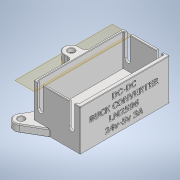
# Autodesk Inventor part: FAN PS CASE
Saved by Autodesk Inventor 2020 (Build 240168000, 168)
## iProperties
Created: 2019-12-23
Part Number: FAN PS CASE
Material: Generic
Document SubType Name: Modeling
Designer: pepd9
Density: 1 g/cm^3
Appearance: Default
Author: pepd9
Autodesk Inventor part; units mm, degrees
(part 1 of 2)
ref_plane "YZ Plane" through (0, 0, 0) normal (1, 0, 0) x (0, 1, 0)
ref_plane "XZ Plane" through (0, 0, 0) normal (0, 1, 0) x (-1, 0, 0)
ref_plane "XY Plane" through (0, 0, 0) normal (0, 0, 1) x (1, 0, 0)
sketch "Sketch1" plane through (0, 0, 0) normal (0, 1, 0) x (-1, 0, 0)
  line L0 (12.5, -25) -> (-12.5, -25)
  line L1 (-12.5, -25) -> (-12.5, 25)
  line L2 (-12.5, 25) -> (12.5, 25)
  line L3 (12.5, 25) -> (12.5, -25)
  line L4 (12.5, -25) -> (-12.5, 25) construction
  line L5 (-12.5, -25) -> (12.5, 25) construction
  line L6 (-12.5, -25) -> (-13.5, -25)
  line L7 (-13.5, -25) -> (-13.5, 25)
  line L8 (-13.5, 25) -> (-12.5, 25)
  line L9 (-12.5, 25) -> (-12.5, -25)
  point P0 (0, 0)
  point P1 (-13, 25)
  dimension "d6" = 25
  dimension "d7" = 50
  dimension "d98" = 1
  constraints: 20 end point, 4 parallel, 3 midpoint, 2 horizontal, 2 perpendicular, 1 horizontal alignment
  measures "d6" distance of L0.start L0.end
  measures "d7" distance of L0.end L1.end
  measures "d98" distance of L7.end L8.end
extrude "Extrusion1" add sketch "Sketch1" along normal blind 5
sketch "Sketch2" plane through (0, 5, 0) normal (0, 1, 0) x (1, 0, 0)
  point P0 (0, 0)
  point P1 (8, 15)
  point P2 (-8, -15)
  dimension "d2" = 30
  dimension "d3" = 16
  dimension "d4" = 8
  dimension "d5" = 15
  measures "d2" vertical distance of point (-8, -15) point (8, 15)
  measures "d3" horizontal distance of point (8, 15) point (-8, -15)
  measures "d4" horizontal distance of point (8, 15) point (0, 0)
  measures "d5" vertical distance of point (0, 0) point (8, 15)
hole "Hole1" at (8, 5, -15) at (-8, 5, 15) direction (0, -1, 0) diameter 3.4 end through all clearance for "Socket Head Cap Screw" size "M3" standard "Ansi Metric M Profile"
sketch "Sketch3" plane through (0, 0, 0) normal (0, -1, 0) x (1, 0, 0)
  circle A0 centre (-8, 15) radius 1.7 projected
  circle A1 centre (8, -15) radius 1.7 projected
  line L0 (-5.25, 13.4123) -> (-8, 11.8246)
  line L1 (-8, 11.8246) -> (-10.75, 13.4123)
  line L2 (-10.75, 13.4123) -> (-10.75, 16.5877)
  line L3 (-10.75, 16.5877) -> (-8, 18.1754)
  line L4 (-8, 18.1754) -> (-5.25, 16.5877)
  line L5 (-5.25, 16.5877) -> (-5.25, 13.4123)
  line L6 (10.75, -16.5877) -> (8, -18.1754)
  line L7 (8, -18.1754) -> (5.25, -16.5877)
  line L8 (5.25, -16.5877) -> (5.25, -13.4123)
  line L9 (5.25, -13.4123) -> (8, -11.8246)
  line L10 (8, -11.8246) -> (10.75, -13.4123)
  line L11 (10.75, -13.4123) -> (10.75, -16.5877)
  point P0 (0, 0)
  dimension "d15" = 5.5
  dimension "d16" = 5.5
  constraints: 24 end point, 2 coincident, 2 vertical, 26 other
  measures "d15" distance between parallel lines of L8 L11
  measures "d16" distance between parallel lines of L2 L5
extrude "Extrusion2" cut sketch "Sketch3" against normal blind 3
sketch "Sketch4" plane through (0, 5, 0) normal (0, 1, 0) x (1, 0, 0)
  circle A0 centre (8, 15) radius 1.7 projected
  circle A1 centre (-8, -15) radius 1.7 projected
  line L0 (-12.5, 25) -> (-12.5, -25) projected
  line L1 (-12.5, -25) -> (13.5, -25) projected
  circle A2 centre (8, 15) radius 1.7 projected
  circle A3 centre (8, 15) radius 3
  circle A4 centre (-8, -15) radius 3
  line L2 (13.5, 25) -> (-12.5, 25) projected
  line L3 (13.5, -25) -> (13.5, 25) projected
  point P0 (0, 0)
  dimension "d19" = 6
  dimension "d20" = 6
  constraints: 2 centre point, 2 coincident
  measures "d19" diameter of A3
  measures "d20" diameter of A4
extrude "Extrusion3" add sketch "Sketch4" along normal blind 4 contours A3 | A4
sketch "Sketch5" plane through (0, 3, 0) normal (0, -1, 0) x (1, 0, 0)
  line L0 (-5.25, 13.4123) -> (-8, 11.8246) projected
  line L1 (-5.25, 16.5877) -> (-5.25, 13.4123) projected
  line L2 (-8, 18.1754) -> (-5.25, 16.5877) projected
  line L3 (-10.75, 16.5877) -> (-8, 18.1754) projected
  line L4 (-10.75, 13.4123) -> (-10.75, 16.5877) projected
  line L5 (-8, 11.8246) -> (-10.75, 13.4123) projected
  circle A0 centre (-8, 15) radius 1.7 projected
  line L6 (10.75, -13.4123) -> (10.75, -16.5877) projected
  line L7 (8, -11.8246) -> (10.75, -13.4123) projected
  line L8 (5.25, -13.4123) -> (8, -11.8246) projected
  line L9 (5.25, -16.5877) -> (5.25, -13.4123) projected
  line L10 (8, -18.1754) -> (5.25, -16.5877) projected
  line L11 (10.75, -16.5877) -> (8, -18.1754) projected
  circle A1 centre (8, -15) radius 1.7 projected
  line L12 (-12.3859, 16.7) -> (-3.6141, 16.7)
  line L13 (-3.6141, 16.7) -> (-3.6141, 13.3)
  line L14 (-3.6141, 13.3) -> (-12.3859, 13.3)
  line L15 (-12.3859, 13.3) -> (-12.3859, 16.7)
  line L16 (-12.3859, 16.7) -> (-3.6141, 13.3) construction
  line L17 (-3.6141, 16.7) -> (-12.3859, 13.3) construction
  line L18 (4.5782, -13.3) -> (11.4218, -13.3)
  line L19 (11.4218, -13.3) -> (11.4218, -16.7)
  line L20 (11.4218, -16.7) -> (4.5782, -16.7)
  line L21 (4.5782, -16.7) -> (4.5782, -13.3)
  line L22 (4.5782, -13.3) -> (11.4218, -16.7) construction
  line L23 (11.4218, -13.3) -> (4.5782, -16.7) construction
  point P0 (0, 0)
  point P1 (5.4445, -16.7)
  point P2 (8, -16.7)
  point P3 (8, -13.3)
  point P4 (5.4445, -13.3)
  point P5 (10.5555, -13.3)
  point P6 (10.5555, -16.7)
  point P7 (-10.5555, 13.3)
  point P8 (-8, 13.3)
  point P9 (-8, 16.7)
  point P10 (-10.5555, 16.7)
  point P11 (-5.4445, 16.7)
  point P12 (-5.4445, 13.3)
  dimension "d23" = 3.4
  dimension "d24" = 3.4
  constraints: 24 end point, 4 midpoint, 4 parallel, 2 horizontal, 2 perpendicular
  measures "d23" distance of L12.end L13.end
  measures "d24" distance of L18.end L19.end
extrude "Extrusion4" cut sketch "Sketch5" against normal blind 0.5 contours L0 L14 A0 L12 L2 L1 | L14 L5 L4 L3 L12 A0 | L6 L11 L20 A1 L18 L7 | A1 L20 L10 L9 L8 L18
sketch "Sketch6" plane through (0, 3.5, 0) normal (0, -1, 0) x (1, 0, 0)
  line L0 (-5.25, 16.5877) -> (-5.25, 13.4123) projected
  line L1 (-5.4445, 16.7) -> (-5.25, 16.5877) projected
  line L2 (-8, 16.7) -> (-5.4445, 16.7) projected
  arc A0 (-8, 13.3) -> (-8, 16.7) centre (-8, 15) ccw projected
  line L3 (-5.4445, 13.3) -> (-8, 13.3) projected
  line L4 (-5.25, 13.4123) -> (-5.4445, 13.3) projected
  line L5 (-10.75, 16.5877) -> (-10.5555, 16.7) projected
  line L6 (-10.75, 13.4123) -> (-10.75, 16.5877) projected
  line L7 (-10.5555, 13.3) -> (-10.75, 13.4123) projected
  line L8 (-8, 13.3) -> (-10.5555, 13.3) projected
  arc A1 (-8, 16.7) -> (-8, 13.3) centre (-8, 15) ccw projected
  line L9 (-10.5555, 16.7) -> (-8, 16.7) projected
  line L10 (10.5555, -13.3) -> (10.75, -13.4123) projected
  line L11 (8, -13.3) -> (10.5555, -13.3) projected
  arc A2 (8, -16.7) -> (8, -13.3) centre (8, -15) ccw projected
  line L12 (10.5555, -16.7) -> (8, -16.7) projected
  line L13 (10.75, -16.5877) -> (10.5555, -16.7) projected
  line L14 (10.75, -13.4123) -> (10.75, -16.5877) projected
  line L15 (5.25, -13.4123) -> (5.4445, -13.3) projected
  line L16 (5.25, -16.5877) -> (5.25, -13.4123) projected
  line L17 (5.4445, -16.7) -> (5.25, -16.5877) projected
  line L18 (8, -16.7) -> (5.4445, -16.7) projected
  arc A3 (8, -13.3) -> (8, -16.7) centre (8, -15) ccw projected
  line L19 (5.4445, -13.3) -> (8, -13.3) projected
  line L20 (6.3, -12.0236) -> (9.7, -12.0236)
  line L21 (9.7, -12.0236) -> (9.7, -17.9764)
  line L22 (9.7, -17.9764) -> (6.3, -17.9764)
  line L23 (6.3, -17.9764) -> (6.3, -12.0236)
  line L24 (6.3, -12.0236) -> (9.7, -17.9764) construction
  line L25 (9.7, -12.0236) -> (6.3, -17.9764) construction
  line L26 (-9.7, 18.2149) -> (-6.3, 18.2149)
  line L27 (-6.3, 18.2149) -> (-6.3, 11.7851)
  line L28 (-6.3, 11.7851) -> (-9.7, 11.7851)
  line L29 (-9.7, 11.7851) -> (-9.7, 18.2149)
  line L30 (-9.7, 18.2149) -> (-6.3, 11.7851) construction
  line L31 (-6.3, 18.2149) -> (-9.7, 11.7851) construction
  point P0 (0, 0)
  point P1 (9.7, -16.7)
  point P2 (9.7, -15)
  point P3 (9.7, -13.3)
  point P4 (6.3, -13.3)
  point P5 (6.3, -15)
  point P6 (6.3, -16.7)
  point P7 (-9.7, 15)
  point P8 (-9.7, 13.3)
  point P9 (-9.7, 16.7)
  point P10 (-6.3, 15)
  point P11 (-6.3, 16.7)
  point P12 (-6.3, 13.3)
  dimension "d27" = 3.4
  dimension "d28" = 3.4
  constraints: 24 end point, 4 midpoint, 4 parallel, 2 horizontal, 2 perpendicular
  measures "d27" distance of L21.end L22.end
  measures "d28" distance of L27.end L28.end
extrude "Extrusion5" cut sketch "Sketch6" against normal blind 0.5 contours L27 A0 L2 | L3 A0 L27 | A1 L29 L9 | L8 L29 A1 | L21 A2 L11 | A3 L23 L19 | L21 L12 A2 | A3 L18 L23
sketch "Sketch7" plane through (0, 5, 0) normal (0, 1, 0) x (1, 0, 0)
  circle A0 centre (-8, -15) radius 3 projected
  circle A1 centre (8, 15) radius 3 projected
  line L0 (-12.5, 25) -> (-12.5, -25) projected
  line L1 (-12.5, -25) -> (13.5, -25) projected
  line L2 (11.3, 23.8) -> (11.3, -23.8)
  line L3 (11.3, -23.8) -> (-11.3, -23.8)
  line L4 (-11.3, -23.8) -> (-11.3, 23.8)
  line L5 (-11.3, 23.8) -> (11.3, 23.8)
  line L6 (13.5, 25) -> (-12.5, 25) projected
  line L7 (13.5, -25) -> (13.5, 25) projected
  point P0 (0, 0)
  constraints: 8 end point, 1 other
extrude "Extrusion6" add sketch "Sketch7" along normal blind 18 contours L6 L7 L1 L0
sketch "Sketch8" plane through (0, 0, 0) normal (0, -1, 0) x (1, 0, 0)
  circle A0 centre (-16.5, 28) radius 4
  circle A1 centre (-16.5, -12) radius 4
  line L0 (-12.5, -25) -> (-12.5, 25) projected
  line L1 (-12.5, 25) -> (13.5, 25) projected
  line L2 (-18.122, -15.6564) -> (-12.5, -18.9022)
  line L3 (-18.122, -8.3436) -> (-12.5, -5.0978)
  line L4 (-19.3561, 25.1995) -> (-12.5, 13.3244)
  line L5 (-14.0743, 31.1806) -> (-3.3692, 25)
  line L6 (-12.5, 25) -> (13.5, 25) projected
  point P0 (0, 0)
  point P1 (12.5, 25)
  point P2 (-12.5, -12)
  dimension "d34" = 8
  dimension "d35" = 8
  dimension "d36" = 4
  dimension "d37" = 40
  dimension "d38" = 3
  dimension "d39" = 60
  dimension "d40" = 60
  dimension "d41" = 30
  dimension "d42" = 30
  constraints: 8 end point, 4 point on circle, 4 point on line, 2 centre point, 1 vertical alignment
  measures "d34" diameter of A0
  measures "d35" diameter of A1
  measures "d36" distance from line of L0 A1.centre
  measures "d37" distance of A0.centre A1.centre
  measures "d38" distance from line of L1 A0.centre
  measures "d39" angle of L0 L2
  measures "d40" angle of L0 L3
  measures "d41" angle of L0 L4
  measures "d42" angle of L1 L5
extrude "Extrusion7" add sketch "Sketch8" against normal blind 4
sketch "Sketch9" plane through (0, 4, 0) normal (0, 1, 0) x (1, 0, 0)
  arc A0 (-18.122, 15.6564) -> (-18.122, 8.3436) centre (-16.5, 12) ccw projected
  arc A1 (-19.3561, -25.1995) -> (-14.0743, -31.1806) centre (-16.5, -28) ccw projected
  point P0 (0, 0)
hole "Hole2" at (-16.5, 4, -12) at (-16.5, 4, 28) direction (0, -1, 0) diameter 3.4 end through all clearance for "Socket Head Cap Screw" size "M3" standard "Ansi Metric M Profile"
sketch "Sketch10" plane through (12.5, 0, -25) normal (0, 0, -1) x (-1, 0, 0)
  line L0 (0, 0) -> (25, 0) projected
  line L1 (25, 0) -> (25, 23) projected
  line L2 (0, 23) -> (25, 23) projected
  line L3 (0, 0) -> (0, 23) projected
  circle A0 centre (3.75, 10.4995) radius 1.5
  circle A1 centre (21.25, 10.4995) radius 1.5
  line L4 (1.2, 23) -> (23.8, 23) projected
  line L5 (2.25, 10.4995) -> (5.25, 10.4995)
  line L6 (5.25, 10.4995) -> (5.25, 23)
  line L7 (5.25, 23) -> (2.25, 23)
  line L8 (2.25, 23) -> (2.25, 10.4995)
  line L9 (22.75, 10.4995) -> (19.75, 10.4995)
  line L10 (19.75, 10.4995) -> (19.75, 23)
  line L11 (19.75, 23) -> (22.75, 23)
  line L12 (22.75, 23) -> (22.75, 10.4995)
  point P0 (12.5, 0)
  point P1 (5.25, 10.4995)
  dimension "d52" = 3
  dimension "d53" = 3
  dimension "d54" = 3
  dimension "d72" = 3.75
  dimension "d73" = 3.75
  constraints: 16 end point, 4 parallel, 2 horizontal, 2 perpendicular, 2 point on line, 6 other
  measures "d54" distance of L10.end L11.end
  measures "d72" distance from line of L3 point (3.75, 10.499)
  measures "d73" distance from line of L1 point (21.25, 10.499)
extrude "Extrusion8" cut sketch "Sketch10" against normal through all contours L2 L6 A0 L8 | L12 A1 L10 L2 | L5 A0 | A0 L5 | L9 A1 | A1 L9
sketch "Sketch11" plane through (0, 0, 0) normal (0, -1, 0) x (1, 0, 0)
  circle A0 centre (-16.5, 0) radius 4
  line L0 (-12.5, -25) -> (-12.5, 25) projected
  line L1 (-12.5, 25) -> (13.5, 25) projected
  line L2 (-16.5, -4) -> (-12.5, -4)
  line L3 (-16.5, 4) -> (-12.5, 4)
  point P0 (0, 0)
  point P1 (-10.25, 25)
  dimension "d57" = 8
  dimension "d58" = 4
  dimension "d59" = 25
  constraints: 4 end point, 2 point on circle, 2 point on line, 2 tangent, 1 centre point, 1 horizontal, 1 perpendicular
  measures "d57" diameter of A0
  measures "d58" distance from line of A0.centre L0
  measures "d59" distance from line of L1 A0.centre
extrude "Extrusion9" add sketch "Sketch11" against normal up to surface (23 mm away)
sketch "Sketch12" plane through (0, 23, 0) normal (0, 1, 0) x (1, 0, 0)
  arc A0 (-16.5, 4) -> (-16.5, -4) centre (-16.5, 0) ccw projected
  point P0 (0, 0)
hole "Hole3" at (-16.5, 23, 0) direction (0, -1, 0) diameter 3.4 end through all clearance for "Socket Head Cap Screw" size "M3" standard "Ansi Metric M Profile"
sketch "Sketch13" plane through (0, 4, 0) normal (0, 1, 0) x (1, 0, 0)
  circle A0 centre (-16.5, 12) radius 1.7 projected
  line L0 (-18.122, 8.3436) -> (-12.5, 5.0978) projected
  line L1 (-12.5, 18.9022) -> (-12.5, 5.0978) projected
  line L2 (-12.5, 18.9022) -> (-18.122, 15.6564) projected
  arc A1 (-18.122, 15.6564) -> (-18.122, 8.3436) centre (-16.5, 12) ccw projected
  circle A2 centre (-16.5, 0) radius 1.7 projected
  line L3 (-12.5, 25) -> (-12.5, 4) projected
  line L4 (-16.5, 4) -> (-12.5, 4) projected
  arc A3 (-16.5, 4) -> (-16.5, -4) centre (-16.5, 0) ccw projected
  line L5 (-12.5, -4) -> (-16.5, -4) projected
  line L6 (-12.5, -4) -> (-12.5, -25) projected
  line L7 (-12.5, -25) -> (-10.25, -25) projected
  line L8 (-10.25, -23.8) -> (-11.3, -23.8) projected
  line L9 (-11.3, -23.8) -> (-11.3, 23.8) projected
  line L10 (-11.3, 23.8) -> (-10.25, 23.8) projected
  arc A4 (-18.122, 15.6564) -> (-18.122, 8.3436) centre (-16.5, 12) ccw projected
  line L11 (-20.5, 12) -> (-20.5, 0)
  line L12 (13.5, -25) -> (13.5, 25) projected
  line L13 (7.25, 25) -> (-7.25, 25) projected
  line L14 (11.3, 23.8) -> (11.3, -23.8) projected
  line L15 (-10.25, 23.8) -> (-10.25, 25) projected
  line L16 (-10.25, 25) -> (-12.5, 25) projected
  line L17 (-10.25, -25) -> (-10.25, -23.8) projected
  line L18 (-7.25, 25) -> (-7.25, 23.8) projected
  line L19 (-7.25, 23.8) -> (7.25, 23.8) projected
  line L20 (7.25, 23.8) -> (7.25, 25) projected
  line L21 (10.25, 25) -> (10.25, 23.8) projected
  line L22 (10.25, 23.8) -> (11.3, 23.8) projected
  line L23 (11.3, -23.8) -> (10.25, -23.8) projected
  line L24 (10.25, -23.8) -> (10.25, -25) projected
  line L25 (10.25, -25) -> (13.5, -25) projected
  line L26 (13.5, 25) -> (10.25, 25) projected
  point P0 (0, 0)
  constraints: 3 point on circle, 2 end point
extrude "Extrusion10" add sketch "Sketch13" against normal up to surface (4 mm away) contours L0 L3 L4 A3 L11 A1
fillet "Fillet1" radius 2 2 edges at (-12.5, 11.5, 4) (-12.5, 13.5, -4)
fillet "Fillet2" radius 0.4 12 edges at (11.3, 14, -23.8) (-11.3, 14, -23.8) (11.3, 14, 23.8) (-11.3, 14, 23.8) (-12.5, 13.5, 25) (-3.3692, 2, 25) (-12.5, 2, 13.3244) (-12.5, 2, -18.9022) (-19.3561, 2, 25.1995) (13.5, 11.5, -25) (-12.5, 11.5, -25) (13.5, 11.5, 25)
chamfer "Chamfer1" distance 0.6 angle 45 12 edges at (5.25, 0, -15) (6.625, 0, -17.3816) (9.375, 0, -17.3816) (10.75, 0, -15) (9.375, 0, -12.6184) (6.625, 0, -12.6184) (-10.75, 0, 15) (-9.375, 0, 12.6184) (-6.625, 0, 12.6184) (-5.25, 0, 15) (-6.625, 0, 17.3816) (-9.375, 0, 17.3816)
chamfer "Chamfer2" distance 0.5 angle 45 10 edges at (-19.4826, 4, 30.6653) (-19.3578, 4, 25.1967) (-15.9425, 4, 19.287) (-12.5136, 4, 13.3208) (-8.7682, 4, 28.1171) (-3.3656, 4, 25.0136) (-20.5, 4, -6) (-19.8532, 4, -14.1808) (-15.411, 4, -17.2216) (-12.5536, 4, -18.9332)
chamfer "Chamfer3" distance 0.25 angle 45 26 edges at (-16.5, 4, -13.7) (-16.5, 4, 26.3) (-20.5, 23, 0) (-15.5, 23, -4) (-13.0858, 23, -4.5858) (-12.5, 23, 15.3) (-12.5, 23, -15.3) (-15.5, 23, 4) (-13.0858, 23, 4.5858) (-12.3828, 23, 24.8828) (-11.175, 23, 25) (-16.5, 23, -1.7) (0, 23, 25) (11.675, 23, 25) (11.3, 23, 0) (11.1828, 23, 23.6828) (10.575, 23, 23.8) (11.1828, 23, -23.6828) (10.575, 23, -23.8) (0, 23, 23.8) (0, 23, -23.8) (-11.3, 23, 0) (-11.1828, 23, -23.6828) (-10.575, 23, -23.8) (-11.1828, 23, 23.6828) (-10.575, 23, 23.8)
ref_plane "Work Plane1" through (0, 20, 0) normal (0, 1, 0) x (1, 0, 0)
sketch "Sketch14" plane through (0, 20, 0) normal (0, 1, 0) x (1, 0, 0)
  circle A0 centre (-16.5, 0) radius 1.7 projected
  line L0 (-19.4, -2.85) -> (-13.6, -2.85)
  line L1 (-13.6, -2.85) -> (-13.6, 2.85)
  line L2 (-13.6, 2.85) -> (-19.4, 2.85)
  line L3 (-19.4, 2.85) -> (-19.4, -2.85)
  line L4 (-19.4, -2.85) -> (-13.6, 2.85) construction
  line L5 (-13.6, -2.85) -> (-19.4, 2.85) construction
  line L6 (-19.4, -2.85) -> (-24.9, -2.85)
  line L7 (-24.9, -2.85) -> (-24.9, 2.85)
  line L8 (-24.9, 2.85) -> (-19.4, 2.85)
  line L9 (-19.4, 2.85) -> (-19.4, -2.85)
  point P0 (0, 0)
  dimension "d85" = 5.8
  dimension "d86" = 5.7
  dimension "d87" = 5.5
  dimension "d88" = 5.7
  constraints: 20 end point, 4 parallel, 2 horizontal, 2 midpoint, 2 perpendicular
  measures "d85" distance of L2.end L1.end
  measures "d86" distance of L1.end L0.end
  measures "d87" distance of L7.end L8.end
  measures "d88" distance of L6.end L7.end
extrude "Extrusion11" cut sketch "Sketch14" against normal blind 1.7
sketch "Sketch15" plane through (0, 20, 0) normal (0, -1, 0) x (1, 0, 0)
  arc A0 (-19.3067, 2.85) -> (-19.3067, -2.85) centre (-16.5, 0) ccw projected
  line L0 (-13.6, -2.85) -> (-19.3067, -2.85) projected
  line L1 (-13.6, 2.85) -> (-13.6, -2.85) projected
  line L2 (-19.3067, 2.85) -> (-13.6, 2.85) projected
  circle A1 centre (-16.5, 0) radius 1.7 projected
  line L3 (-14.8283, -3.0472) -> (-18.2283, -3.0472)
  line L4 (-18.2283, -3.0472) -> (-18.2283, 3.0472)
  line L5 (-18.2283, 3.0472) -> (-14.8283, 3.0472)
  line L6 (-14.8283, 3.0472) -> (-14.8283, -3.0472)
  line L7 (-14.8283, -3.0472) -> (-18.2283, 3.0472) construction
  line L8 (-18.2283, -3.0472) -> (-14.8283, 3.0472) construction
  point P0 (0, 0)
  point P1 (-16.5283, 0)
  point P2 (-14.8283, -2.85)
  point P3 (-14.8283, -0.3088)
  point P4 (-14.8283, 0.3088)
  point P5 (-14.8283, 2.85)
  point P6 (-18.2283, 2.85)
  point P7 (-18.2283, -2.85)
  dimension "d91" = 3.4
  constraints: 12 end point, 2 midpoint, 2 parallel, 1 horizontal, 1 perpendicular
  measures "d91" distance of L4.end L5.end
extrude "Extrusion12" cut sketch "Sketch15" against normal blind 0.5 contours L2 L6 A1 L0 L4
sketch "Sketch16" plane through (0, 20.5, 0) normal (0, -1, 0) x (1, 0, 0)
  arc A0 (-14.8283, 0.3088) -> (-14.8283, -0.3088) centre (-16.5, 0) ccw projected
  line L0 (-14.8, -1.7) -> (-18.2, -1.7)
  line L1 (-18.2, -1.7) -> (-18.2, 1.7)
  line L2 (-18.2, 1.7) -> (-14.8, 1.7)
  line L3 (-14.8, 1.7) -> (-14.8, -1.7)
  line L4 (-14.8, -1.7) -> (-18.2, 1.7) construction
  line L5 (-18.2, -1.7) -> (-14.8, 1.7) construction
  circle A1 centre (-16.5, 0) radius 1.7 projected
  point P0 (0, 0)
  point P1 (-14.8, 0)
  point P2 (-16.5, 1.7)
  point P3 (-16.5, -1.7)
  point P4 (-18.2, 0)
  dimension "d94" = 3.4
  dimension "d95" = 3.4
  constraints: 12 end point, 2 midpoint, 2 parallel, 1 horizontal, 1 perpendicular
  measures "d94" distance of L1.end L2.end
  measures "d95" distance of L0.end L1.end
extrude "Extrusion13" cut sketch "Sketch16" against normal blind 0.5 contours A0 L2 L3 A1 | A0 L1 L2 | L3 L0 A0 A1 | A0 L0 L1
sketch "Sketch17" plane through (13.5, 0.25, 24.6) normal (1, 0, 0) x (0, 0, -1)
  line L0 (4.6127, 20.5668) -> (43.452, 20.5668) construction
  line L1 (43.452, 20.5668) -> (43.452, 2.328) construction
  line L2 (43.452, 2.328) -> (4.6127, 2.328) construction
  line L3 (4.6127, 2.328) -> (4.6127, 20.5668) construction
  spline S0 degree 2 poles (20.189, 18.98) (20.189, 18.5524) (19.8158, 17.8801) (19.5315, 17.6997) knots 0 0 0 1 2 2 2
  spline S1 degree 2 poles (19.5315, 17.6997) (19.2942, 17.5465) (18.7356, 17.4575) (18.4217, 17.4575) knots 0 0 0 1 2 2 2
  line L4 (18.4217, 17.4575) -> (17.4677, 17.4575)
  line L5 (17.4677, 17.4575) -> (17.4677, 20.5075)
  line L6 (17.4677, 20.5075) -> (18.4119, 20.5075)
  spline S2 degree 2 poles (18.4119, 20.5075) (18.7332, 20.5075) (19.2942, 20.4259) (19.5414, 20.2677) knots 0 0 0 1 2 2 2
  spline S3 degree 2 poles (19.5414, 20.2677) (19.8405, 20.0749) (20.189, 19.4224) (20.189, 18.98) knots 0 0 0 1 2 2 2
  spline S4 degree 2 poles (19.403, 18.985) (19.403, 19.2865) (19.1954, 19.7166) (18.9828, 19.8377) knots 0 0 0 1 2 2 2
  spline S5 degree 2 poles (18.9828, 19.8377) (18.8271, 19.9217) (18.486, 19.939) (18.2487, 19.939) knots 0 0 0 1 2 2 2
  line L7 (18.2487, 19.939) -> (18.2339, 19.939)
  line L8 (18.2339, 19.939) -> (18.2339, 18.0284)
  line L9 (18.2339, 18.0284) -> (18.2487, 18.0284)
  spline S6 degree 2 poles (18.2487, 18.0284) (18.5058, 18.0284) (18.8592, 18.0457) (19.0199, 18.1471) knots 0 0 0 1 2 2 2
  spline S7 degree 2 poles (19.0199, 18.1471) (19.2077, 18.2657) (19.403, 18.6834) (19.403, 18.985) knots 0 0 0 1 2 2 2
  spline S8 degree 2 poles (21.9587, 17.3982) (21.2715, 17.3982) (20.4658, 18.2286) (20.4658, 18.98) knots 0 0 0 1 2 2 2
  spline S9 degree 2 poles (20.4658, 18.98) (20.4658, 19.7042) (21.274, 20.5668) (21.9611, 20.5668) knots 0 0 0 1 2 2 2
  spline S10 degree 2 poles (21.9611, 20.5668) (22.1416, 20.5668) (22.4332, 20.5248) (22.5667, 20.4902) knots 0 0 0 1 2 2 2
  spline S11 degree 2 poles (22.5667, 20.4902) (22.6705, 20.4581) (22.9152, 20.3518) (22.9918, 20.3122) knots 0 0 0 1 2 2 2
  line L10 (22.9918, 20.3122) -> (22.9918, 19.5856)
  line L11 (22.9918, 19.5856) -> (22.9152, 19.5856)
  spline S12 degree 2 poles (22.9152, 19.5856) (22.8583, 19.635) (22.6903, 19.7734) (22.584, 19.8377) knots 0 0 0 1 2 2 2
  spline S13 degree 2 poles (22.584, 19.8377) (22.4777, 19.9044) (22.2231, 19.9959) (22.0822, 19.9959) knots 0 0 0 1 2 2 2
  spline S14 degree 2 poles (22.0822, 19.9959) (21.9166, 19.9959) (21.6423, 19.892) (21.5162, 19.761) knots 0 0 0 1 2 2 2
  spline S15 degree 2 poles (21.5162, 19.761) (21.4025, 19.6449) (21.2567, 19.2469) (21.2567, 18.9775) knots 0 0 0 1 2 2 2
  spline S16 degree 2 poles (21.2567, 18.9775) (21.2567, 18.6933) (21.4075, 18.3053) (21.5311, 18.1866) knots 0 0 0 1 2 2 2
  spline S17 degree 2 poles (21.5311, 18.1866) (21.6497, 18.0704) (21.9414, 17.9691) (22.0872, 17.9691) knots 0 0 0 1 2 2 2
  spline S18 degree 2 poles (22.0872, 17.9691) (22.238, 17.9691) (22.5123, 18.0704) (22.6062, 18.1322) knots 0 0 0 1 2 2 2
  spline S19 degree 2 poles (22.6062, 18.1322) (22.71, 18.194) (22.8658, 18.325) (22.9226, 18.3769) knots 0 0 0 1 2 2 2
  line L12 (22.9226, 18.3769) -> (22.9918, 18.3769)
  line L13 (22.9918, 18.3769) -> (22.9918, 17.6602)
  spline S20 degree 2 poles (22.9918, 17.6602) (22.9078, 17.6206) (22.6878, 17.5217) (22.5692, 17.4871) knots 0 0 0 1 2 2 2
  spline S21 degree 2 poles (22.5692, 17.4871) (22.4258, 17.4427) (22.1762, 17.3982) (21.9587, 17.3982) knots 0 0 0 1 2 2 2
  line L14 (24.7096, 18.5203) -> (23.3527, 18.5203)
  line L15 (23.3527, 18.5203) -> (23.3527, 19.0888)
  line L16 (23.3527, 19.0888) -> (24.7096, 19.0888)
  line L17 (24.7096, 19.0888) -> (24.7096, 18.5203)
  spline S22 degree 2 poles (27.9746, 18.98) (27.9746, 18.5524) (27.6014, 17.8801) (27.3172, 17.6997) knots 0 0 0 1 2 2 2
  spline S23 degree 2 poles (27.3172, 17.6997) (27.0799, 17.5465) (26.5213, 17.4575) (26.2074, 17.4575) knots 0 0 0 1 2 2 2
  line L18 (26.2074, 17.4575) -> (25.2534, 17.4575)
  line L19 (25.2534, 17.4575) -> (25.2534, 20.5075)
  line L20 (25.2534, 20.5075) -> (26.1975, 20.5075)
  spline S24 degree 2 poles (26.1975, 20.5075) (26.5188, 20.5075) (27.0799, 20.4259) (27.3271, 20.2677) knots 0 0 0 1 2 2 2
  spline S25 degree 2 poles (27.3271, 20.2677) (27.6261, 20.0749) (27.9746, 19.4224) (27.9746, 18.98) knots 0 0 0 1 2 2 2
  spline S26 degree 2 poles (27.1886, 18.985) (27.1886, 19.2865) (26.981, 19.7166) (26.7685, 19.8377) knots 0 0 0 1 2 2 2
  spline S27 degree 2 poles (26.7685, 19.8377) (26.6128, 19.9217) (26.2717, 19.939) (26.0344, 19.939) knots 0 0 0 1 2 2 2
  line L21 (26.0344, 19.939) -> (26.0196, 19.939)
  line L22 (26.0196, 19.939) -> (26.0196, 18.0284)
  line L23 (26.0196, 18.0284) -> (26.0344, 18.0284)
  spline S28 degree 2 poles (26.0344, 18.0284) (26.2914, 18.0284) (26.6449, 18.0457) (26.8055, 18.1471) knots 0 0 0 1 2 2 2
  spline S29 degree 2 poles (26.8055, 18.1471) (26.9934, 18.2657) (27.1886, 18.6834) (27.1886, 18.985) knots 0 0 0 1 2 2 2
  spline S30 degree 2 poles (29.7443, 17.3982) (29.0572, 17.3982) (28.2514, 18.2286) (28.2514, 18.98) knots 0 0 0 1 2 2 2
  spline S31 degree 2 poles (28.2514, 18.98) (28.2514, 19.7042) (29.0597, 20.5668) (29.7468, 20.5668) knots 0 0 0 1 2 2 2
  spline S32 degree 2 poles (29.7468, 20.5668) (29.9272, 20.5668) (30.2189, 20.5248) (30.3523, 20.4902) knots 0 0 0 1 2 2 2
  spline S33 degree 2 poles (30.3523, 20.4902) (30.4561, 20.4581) (30.7008, 20.3518) (30.7775, 20.3122) knots 0 0 0 1 2 2 2
  line L24 (30.7775, 20.3122) -> (30.7775, 19.5856)
  line L25 (30.7775, 19.5856) -> (30.7008, 19.5856)
  spline S34 degree 2 poles (30.7008, 19.5856) (30.644, 19.635) (30.4759, 19.7734) (30.3696, 19.8377) knots 0 0 0 1 2 2 2
  spline S35 degree 2 poles (30.3696, 19.8377) (30.2634, 19.9044) (30.0088, 19.9959) (29.8679, 19.9959) knots 0 0 0 1 2 2 2
  spline S36 degree 2 poles (29.8679, 19.9959) (29.7023, 19.9959) (29.4279, 19.892) (29.3019, 19.761) knots 0 0 0 1 2 2 2
  spline S37 degree 2 poles (29.3019, 19.761) (29.1882, 19.6449) (29.0424, 19.2469) (29.0424, 18.9775) knots 0 0 0 1 2 2 2
  spline S38 degree 2 poles (29.0424, 18.9775) (29.0424, 18.6933) (29.1931, 18.3053) (29.3167, 18.1866) knots 0 0 0 1 2 2 2
  spline S39 degree 2 poles (29.3167, 18.1866) (29.4354, 18.0704) (29.727, 17.9691) (29.8728, 17.9691) knots 0 0 0 1 2 2 2
  spline S40 degree 2 poles (29.8728, 17.9691) (30.0236, 17.9691) (30.298, 18.0704) (30.3919, 18.1322) knots 0 0 0 1 2 2 2
  spline S41 degree 2 poles (30.3919, 18.1322) (30.4957, 18.194) (30.6514, 18.325) (30.7083, 18.3769) knots 0 0 0 1 2 2 2
  line L26 (30.7083, 18.3769) -> (30.7775, 18.3769)
  line L27 (30.7775, 18.3769) -> (30.7775, 17.6602)
  spline S42 degree 2 poles (30.7775, 17.6602) (30.6934, 17.6206) (30.4735, 17.5217) (30.3548, 17.4871) knots 0 0 0 1 2 2 2
  spline S43 degree 2 poles (30.3548, 17.4871) (30.2115, 17.4427) (29.9618, 17.3982) (29.7443, 17.3982) knots 0 0 0 1 2 2 2
  spline S44 degree 2 poles (7.3661, 13.37) (7.3661, 13.1426) (7.1931, 12.7991) (7.0497, 12.6854) knots 0 0 0 1 2 2 2
  spline S45 degree 2 poles (7.0497, 12.6854) (6.8767, 12.5494) (6.4664, 12.4357) (6.1476, 12.4357) knots 0 0 0 1 2 2 2
  line L28 (6.1476, 12.4357) -> (4.9291, 12.4357)
  line L29 (4.9291, 12.4357) -> (4.9291, 15.4857)
  line L30 (4.9291, 15.4857) -> (6.0042, 15.4857)
  spline S46 degree 2 poles (6.0042, 15.4857) (6.3404, 15.4857) (6.6864, 15.4338) (6.8372, 15.3523) knots 0 0 0 1 2 2 2
  spline S47 degree 2 poles (6.8372, 15.3523) (7.0028, 15.2658) (7.1634, 14.9692) (7.1634, 14.7764) knots 0 0 0 1 2 2 2
  spline S48 degree 2 poles (7.1634, 14.7764) (7.1634, 14.5539) (6.941, 14.2054) (6.7433, 14.1239) knots 0 0 0 1 2 2 2
  line L31 (6.7433, 14.1239) -> (6.7433, 14.109)
  spline S49 degree 2 poles (6.7433, 14.109) (7.0275, 14.0497) (7.3661, 13.6814) (7.3661, 13.37) knots 0 0 0 1 2 2 2
  spline S50 degree 2 poles (6.5752, 13.3824) (6.5752, 13.5257) (6.4615, 13.6864) (6.3478, 13.7284) knots 0 0 0 1 2 2 2
  spline S51 degree 2 poles (6.3478, 13.7284) (6.2786, 13.7556) (6.0339, 13.7605) (5.8312, 13.7605) knots 0 0 0 1 2 2 2
  line L32 (5.8312, 13.7605) -> (5.6903, 13.7605)
  line L33 (5.6903, 13.7605) -> (5.6903, 12.9919)
  line L34 (5.6903, 12.9919) -> (5.7324, 12.9919)
  spline S52 degree 2 poles (5.7324, 12.9919) (6.029, 12.9919) (6.2564, 12.9993) (6.375, 13.0512) knots 0 0 0 1 2 2 2
  spline S53 degree 2 poles (6.375, 13.0512) (6.4788, 13.0981) (6.5752, 13.2712) (6.5752, 13.3824) knots 0 0 0 1 2 2 2
  spline S54 degree 2 poles (6.3849, 14.6256) (6.3849, 14.6998) (6.3083, 14.8555) (6.2292, 14.8901) knots 0 0 0 1 2 2 2
  spline S55 degree 2 poles (6.2292, 14.8901) (6.155, 14.9247) (5.9474, 14.9296) (5.7423, 14.9296) knots 0 0 0 1 2 2 2
  line L35 (5.7423, 14.9296) -> (5.6903, 14.9296)
  line L36 (5.6903, 14.9296) -> (5.6903, 14.2821)
  line L37 (5.6903, 14.2821) -> (5.7867, 14.2821)
  spline S56 degree 2 poles (5.7867, 14.2821) (5.982, 14.2821) (6.1402, 14.2895) (6.2242, 14.329) knots 0 0 0 1 2 2 2
  spline S57 degree 2 poles (6.2242, 14.329) (6.3157, 14.3735) (6.3849, 14.5243) (6.3849, 14.6256) knots 0 0 0 1 2 2 2
  spline S58 degree 2 poles (9.0394, 12.3715) (8.424, 12.3715) (7.7616, 12.9647) (7.7616, 13.5381) knots 0 0 0 1 2 2 2
  line L38 (7.7616, 13.5381) -> (7.7616, 15.4857)
  line L39 (7.7616, 15.4857) -> (8.5278, 15.4857)
  line L40 (8.5278, 15.4857) -> (8.5278, 13.5826)
  spline S59 degree 2 poles (8.5278, 13.5826) (8.5278, 13.2637) (8.7675, 12.9523) (9.0394, 12.9523) knots 0 0 0 1 2 2 2
  spline S60 degree 2 poles (9.0394, 12.9523) (9.3039, 12.9523) (9.551, 13.2514) (9.551, 13.5826) knots 0 0 0 1 2 2 2
  line L41 (9.551, 13.5826) -> (9.551, 15.4857)
  line L42 (9.551, 15.4857) -> (10.3173, 15.4857)
  line L43 (10.3173, 15.4857) -> (10.3173, 13.5406)
  spline S61 degree 2 poles (10.3173, 13.5406) (10.3173, 12.977) (9.6722, 12.3715) (9.0394, 12.3715) knots 0 0 0 1 2 2 2
  spline S62 degree 2 poles (12.2204, 12.3764) (11.5333, 12.3764) (10.7275, 13.2069) (10.7275, 13.9583) knots 0 0 0 1 2 2 2
  spline S63 degree 2 poles (10.7275, 13.9583) (10.7275, 14.6825) (11.5358, 15.5451) (12.2229, 15.5451) knots 0 0 0 1 2 2 2
  spline S64 degree 2 poles (12.2229, 15.5451) (12.4033, 15.5451) (12.695, 15.503) (12.8284, 15.4684) knots 0 0 0 1 2 2 2
  spline S65 degree 2 poles (12.8284, 15.4684) (12.9322, 15.4363) (13.1769, 15.33) (13.2536, 15.2905) knots 0 0 0 1 2 2 2
  line L44 (13.2536, 15.2905) -> (13.2536, 14.5638)
  line L45 (13.2536, 14.5638) -> (13.1769, 14.5638)
  spline S66 degree 2 poles (13.1769, 14.5638) (13.1201, 14.6133) (12.952, 14.7517) (12.8457, 14.8159) knots 0 0 0 1 2 2 2
  spline S67 degree 2 poles (12.8457, 14.8159) (12.7395, 14.8827) (12.4849, 14.9741) (12.344, 14.9741) knots 0 0 0 1 2 2 2
  spline S68 degree 2 poles (12.344, 14.9741) (12.1784, 14.9741) (11.904, 14.8703) (11.778, 14.7393) knots 0 0 0 1 2 2 2
  spline S69 degree 2 poles (11.778, 14.7393) (11.6643, 14.6231) (11.5185, 14.2252) (11.5185, 13.9558) knots 0 0 0 1 2 2 2
  spline S70 degree 2 poles (11.5185, 13.9558) (11.5185, 13.6716) (11.6692, 13.2835) (11.7928, 13.1649) knots 0 0 0 1 2 2 2
  spline S71 degree 2 poles (11.7928, 13.1649) (11.9115, 13.0487) (12.2031, 12.9474) (12.3489, 12.9474) knots 0 0 0 1 2 2 2
  spline S72 degree 2 poles (12.3489, 12.9474) (12.4997, 12.9474) (12.7741, 13.0487) (12.868, 13.1105) knots 0 0 0 1 2 2 2
  spline S73 degree 2 poles (12.868, 13.1105) (12.9718, 13.1723) (13.1275, 13.3033) (13.1843, 13.3552) knots 0 0 0 1 2 2 2
  line L46 (13.1843, 13.3552) -> (13.2536, 13.3552)
  line L47 (13.2536, 13.3552) -> (13.2536, 12.6384)
  spline S74 degree 2 poles (13.2536, 12.6384) (13.1695, 12.5989) (12.9495, 12.5) (12.8309, 12.4654) knots 0 0 0 1 2 2 2
  spline S75 degree 2 poles (12.8309, 12.4654) (12.6876, 12.4209) (12.4379, 12.3764) (12.2204, 12.3764) knots 0 0 0 1 2 2 2
  line L48 (16.3777, 12.4357) -> (15.4508, 12.4357)
  line L49 (15.4508, 12.4357) -> (14.6228, 13.674)
  line L50 (14.6228, 13.674) -> (14.4721, 13.4664)
  line L51 (14.4721, 13.4664) -> (14.4721, 12.4357)
  line L52 (14.4721, 12.4357) -> (13.7059, 12.4357)
  line L53 (13.7059, 12.4357) -> (13.7059, 15.4857)
  line L54 (13.7059, 15.4857) -> (14.4721, 15.4857)
  line L55 (14.4721, 15.4857) -> (14.4721, 14.1239)
  line L56 (14.4721, 14.1239) -> (15.4508, 15.4857)
  line L57 (15.4508, 15.4857) -> (16.3332, 15.4857)
  line L58 (16.3332, 15.4857) -> (15.2457, 14.0695)
  line L59 (15.2457, 14.0695) -> (16.3777, 12.4357)
  spline S76 degree 2 poles (19.1707, 12.3764) (18.4835, 12.3764) (17.6778, 13.2069) (17.6778, 13.9583) knots 0 0 0 1 2 2 2
  spline S77 degree 2 poles (17.6778, 13.9583) (17.6778, 14.6825) (18.486, 15.5451) (19.1731, 15.5451) knots 0 0 0 1 2 2 2
  spline S78 degree 2 poles (19.1731, 15.5451) (19.3536, 15.5451) (19.6452, 15.503) (19.7787, 15.4684) knots 0 0 0 1 2 2 2
  spline S79 degree 2 poles (19.7787, 15.4684) (19.8825, 15.4363) (20.1272, 15.33) (20.2038, 15.2905) knots 0 0 0 1 2 2 2
  line L60 (20.2038, 15.2905) -> (20.2038, 14.5638)
  line L61 (20.2038, 14.5638) -> (20.1272, 14.5638)
  spline S80 degree 2 poles (20.1272, 14.5638) (20.0703, 14.6133) (19.9023, 14.7517) (19.796, 14.8159) knots 0 0 0 1 2 2 2
  spline S81 degree 2 poles (19.796, 14.8159) (19.6897, 14.8827) (19.4351, 14.9741) (19.2942, 14.9741) knots 0 0 0 1 2 2 2
  spline S82 degree 2 poles (19.2942, 14.9741) (19.1286, 14.9741) (18.8543, 14.8703) (18.7282, 14.7393) knots 0 0 0 1 2 2 2
  spline S83 degree 2 poles (18.7282, 14.7393) (18.6145, 14.6231) (18.4687, 14.2252) (18.4687, 13.9558) knots 0 0 0 1 2 2 2
  spline S84 degree 2 poles (18.4687, 13.9558) (18.4687, 13.6716) (18.6195, 13.2835) (18.7431, 13.1649) knots 0 0 0 1 2 2 2
  spline S85 degree 2 poles (18.7431, 13.1649) (18.8617, 13.0487) (19.1534, 12.9474) (19.2992, 12.9474) knots 0 0 0 1 2 2 2
  spline S86 degree 2 poles (19.2992, 12.9474) (19.4499, 12.9474) (19.7243, 13.0487) (19.8182, 13.1105) knots 0 0 0 1 2 2 2
  spline S87 degree 2 poles (19.8182, 13.1105) (19.922, 13.1723) (20.0777, 13.3033) (20.1346, 13.3552) knots 0 0 0 1 2 2 2
  line L62 (20.1346, 13.3552) -> (20.2038, 13.3552)
  line L63 (20.2038, 13.3552) -> (20.2038, 12.6384)
  spline S88 degree 2 poles (20.2038, 12.6384) (20.1198, 12.5989) (19.8998, 12.5) (19.7811, 12.4654) knots 0 0 0 1 2 2 2
  spline S89 degree 2 poles (19.7811, 12.4654) (19.6378, 12.4209) (19.3882, 12.3764) (19.1707, 12.3764) knots 0 0 0 1 2 2 2
  spline S90 degree 2 poles (23.4318, 13.9607) (23.4318, 13.2192) (22.6408, 12.3715) (21.9537, 12.3715) knots 0 0 0 1 2 2 2
  spline S91 degree 2 poles (21.9537, 12.3715) (21.2641, 12.3715) (20.4782, 13.2291) (20.4782, 13.9607) knots 0 0 0 1 2 2 2
  spline S92 degree 2 poles (20.4782, 13.9607) (20.4782, 14.6948) (21.2641, 15.55) (21.9537, 15.55) knots 0 0 0 1 2 2 2
  spline S93 degree 2 poles (21.9537, 15.55) (22.6408, 15.55) (23.4318, 14.6998) (23.4318, 13.9607) knots 0 0 0 1 2 2 2
  spline S94 degree 2 poles (22.6408, 13.9607) (22.6408, 14.2351) (22.5296, 14.6182) (22.4332, 14.7393) knots 0 0 0 1 2 2 2
  spline S95 degree 2 poles (22.4332, 14.7393) (22.3368, 14.8654) (22.0897, 14.9741) (21.9562, 14.9741) knots 0 0 0 1 2 2 2
  spline S96 degree 2 poles (21.9562, 14.9741) (21.8153, 14.9741) (21.5854, 14.8728) (21.4792, 14.7442) knots 0 0 0 1 2 2 2
  spline S97 degree 2 poles (21.4792, 14.7442) (21.3852, 14.6256) (21.2691, 14.2326) (21.2691, 13.9607) knots 0 0 0 1 2 2 2
  spline S98 degree 2 poles (21.2691, 13.9607) (21.2691, 13.679) (21.3803, 13.3082) (21.4767, 13.1822) knots 0 0 0 1 2 2 2
  spline S99 degree 2 poles (21.4767, 13.1822) (21.5731, 13.0561) (21.8227, 12.9474) (21.9562, 12.9474) knots 0 0 0 1 2 2 2
  spline S100 degree 2 poles (21.9562, 12.9474) (22.0921, 12.9474) (22.3442, 13.0635) (22.4357, 13.1871) knots 0 0 0 1 2 2 2
  spline S101 degree 2 poles (22.4357, 13.1871) (22.5346, 13.3206) (22.6408, 13.674) (22.6408, 13.9607) knots 0 0 0 1 2 2 2
  line L64 (26.4991, 12.4357) -> (25.7625, 12.4357)
  line L65 (25.7625, 12.4357) -> (24.586, 14.5613)
  line L66 (24.586, 14.5613) -> (24.586, 12.4357)
  line L67 (24.586, 12.4357) -> (23.8865, 12.4357)
  line L68 (23.8865, 12.4357) -> (23.8865, 15.4857)
  line L69 (23.8865, 15.4857) -> (24.8258, 15.4857)
  line L70 (24.8258, 15.4857) -> (25.7996, 13.7383)
  line L71 (25.7996, 13.7383) -> (25.7996, 15.4857)
  line L72 (25.7996, 15.4857) -> (26.4991, 15.4857)
  line L73 (26.4991, 15.4857) -> (26.4991, 12.4357)
  line L74 (29.6652, 15.4857) -> (28.6173, 12.4357)
  line L75 (28.6173, 12.4357) -> (27.8189, 12.4357)
  line L76 (27.8189, 12.4357) -> (26.7709, 15.4857)
  line L77 (26.7709, 15.4857) -> (27.5643, 15.4857)
  line L78 (27.5643, 15.4857) -> (28.2292, 13.417)
  line L79 (28.2292, 13.417) -> (28.8916, 15.4857)
  line L80 (28.8916, 15.4857) -> (29.6652, 15.4857)
  line L81 (29.9495, 12.4357) -> (29.9495, 15.4857)
  line L82 (29.9495, 15.4857) -> (32.0108, 15.4857)
  line L83 (32.0108, 15.4857) -> (32.0108, 14.9049)
  line L84 (32.0108, 14.9049) -> (30.7107, 14.9049)
  line L85 (30.7107, 14.9049) -> (30.7107, 14.3686)
  line L86 (30.7107, 14.3686) -> (31.9095, 14.3686)
  line L87 (31.9095, 14.3686) -> (31.9095, 13.7877)
  line L88 (31.9095, 13.7877) -> (30.7107, 13.7877)
  line L89 (30.7107, 13.7877) -> (30.7107, 13.0166)
  line L90 (30.7107, 13.0166) -> (32.0108, 13.0166)
  line L91 (32.0108, 13.0166) -> (32.0108, 12.4357)
  line L92 (32.0108, 12.4357) -> (29.9495, 12.4357)
  line L93 (35.3475, 12.4357) -> (34.4157, 12.4357)
  line L94 (34.4157, 12.4357) -> (33.5679, 13.5554)
  line L95 (33.5679, 13.5554) -> (33.2911, 13.5554)
  line L96 (33.2911, 13.5554) -> (33.2911, 12.4357)
  line L97 (33.2911, 12.4357) -> (32.5299, 12.4357)
  line L98 (32.5299, 12.4357) -> (32.5299, 15.4857)
  line L99 (32.5299, 15.4857) -> (33.7558, 15.4857)
  spline S102 degree 2 poles (33.7558, 15.4857) (34.0104, 15.4857) (34.3861, 15.4215) (34.5467, 15.3226) knots 0 0 0 1 2 2 2
  spline S103 degree 2 poles (34.5467, 15.3226) (34.7098, 15.2188) (34.9026, 14.895) (34.9026, 14.6479) knots 0 0 0 1 2 2 2
  spline S104 degree 2 poles (34.9026, 14.6479) (34.9026, 14.2994) (34.5863, 13.8619) (34.3218, 13.7333) knots 0 0 0 1 2 2 2
  line L100 (34.3218, 13.7333) -> (35.3475, 12.4357)
  spline S105 degree 2 poles (34.1166, 14.5515) (34.1166, 14.6676) (34.0277, 14.8332) (33.9263, 14.8777) knots 0 0 0 1 2 2 2
  spline S106 degree 2 poles (33.9263, 14.8777) (33.8546, 14.9074) (33.6792, 14.9247) (33.5482, 14.9247) knots 0 0 0 1 2 2 2
  line L101 (33.5482, 14.9247) -> (33.2911, 14.9247)
  line L102 (33.2911, 14.9247) -> (33.2911, 14.1041)
  line L103 (33.2911, 14.1041) -> (33.5111, 14.1041)
  spline S107 degree 2 poles (33.5111, 14.1041) (33.6693, 14.1041) (33.8942, 14.1436) (33.9708, 14.2054) knots 0 0 0 1 2 2 2
  spline S108 degree 2 poles (33.9708, 14.2054) (34.045, 14.2648) (34.1166, 14.4229) (34.1166, 14.5515) knots 0 0 0 1 2 2 2
  line L104 (36.1607, 12.4357) -> (36.1607, 14.9049)
  line L105 (36.1607, 14.9049) -> (35.2585, 14.9049)
  line L106 (35.2585, 14.9049) -> (35.2585, 15.4857)
  line L107 (35.2585, 15.4857) -> (37.829, 15.4857)
  line L108 (37.829, 15.4857) -> (37.829, 14.9049)
  line L109 (37.829, 14.9049) -> (36.9269, 14.9049)
  line L110 (36.9269, 14.9049) -> (36.9269, 12.4357)
  line L111 (36.9269, 12.4357) -> (36.1607, 12.4357)
  line L112 (38.1429, 12.4357) -> (38.1429, 15.4857)
  line L113 (38.1429, 15.4857) -> (40.2043, 15.4857)
  line L114 (40.2043, 15.4857) -> (40.2043, 14.9049)
  line L115 (40.2043, 14.9049) -> (38.9042, 14.9049)
  line L116 (38.9042, 14.9049) -> (38.9042, 14.3686)
  line L117 (38.9042, 14.3686) -> (40.1029, 14.3686)
  line L118 (40.1029, 14.3686) -> (40.1029, 13.7877)
  line L119 (40.1029, 13.7877) -> (38.9042, 13.7877)
  line L120 (38.9042, 13.7877) -> (38.9042, 13.0166)
  line L121 (38.9042, 13.0166) -> (40.2043, 13.0166)
  line L122 (40.2043, 13.0166) -> (40.2043, 12.4357)
  line L123 (40.2043, 12.4357) -> (38.1429, 12.4357)
  line L124 (43.541, 12.4357) -> (42.6092, 12.4357)
  line L125 (42.6092, 12.4357) -> (41.7614, 13.5554)
  line L126 (41.7614, 13.5554) -> (41.4846, 13.5554)
  line L127 (41.4846, 13.5554) -> (41.4846, 12.4357)
  line L128 (41.4846, 12.4357) -> (40.7233, 12.4357)
  line L129 (40.7233, 12.4357) -> (40.7233, 15.4857)
  line L130 (40.7233, 15.4857) -> (41.9493, 15.4857)
  spline S109 degree 2 poles (41.9493, 15.4857) (42.2038, 15.4857) (42.5795, 15.4215) (42.7402, 15.3226) knots 0 0 0 1 2 2 2
  spline S110 degree 2 poles (42.7402, 15.3226) (42.9033, 15.2188) (43.0961, 14.895) (43.0961, 14.6479) knots 0 0 0 1 2 2 2
  spline S111 degree 2 poles (43.0961, 14.6479) (43.0961, 14.2994) (42.7797, 13.8619) (42.5153, 13.7333) knots 0 0 0 1 2 2 2
  line L131 (42.5153, 13.7333) -> (43.541, 12.4357)
  spline S112 degree 2 poles (42.3101, 14.5515) (42.3101, 14.6676) (42.2211, 14.8332) (42.1198, 14.8777) knots 0 0 0 1 2 2 2
  spline S113 degree 2 poles (42.1198, 14.8777) (42.0481, 14.9074) (41.8726, 14.9247) (41.7416, 14.9247) knots 0 0 0 1 2 2 2
  line L132 (41.7416, 14.9247) -> (41.4846, 14.9247)
  line L133 (41.4846, 14.9247) -> (41.4846, 14.1041)
  line L134 (41.4846, 14.1041) -> (41.7046, 14.1041)
  spline S114 degree 2 poles (41.7046, 14.1041) (41.8628, 14.1041) (42.0877, 14.1436) (42.1643, 14.2054) knots 0 0 0 1 2 2 2
  spline S115 degree 2 poles (42.1643, 14.2054) (42.2384, 14.2648) (42.3101, 14.4229) (42.3101, 14.5515) knots 0 0 0 1 2 2 2
  line L135 (17.9657, 7.414) -> (15.9316, 7.414)
  line L136 (15.9316, 7.414) -> (15.9316, 10.464)
  line L137 (15.9316, 10.464) -> (16.6978, 10.464)
  line L138 (16.6978, 10.464) -> (16.6978, 7.9948)
  line L139 (16.6978, 7.9948) -> (17.9657, 7.9948)
  line L140 (17.9657, 7.9948) -> (17.9657, 7.414)
  line L141 (21.4458, 7.414) -> (20.6845, 7.414)
  line L142 (20.6845, 7.414) -> (20.6845, 9.4358)
  line L143 (20.6845, 9.4358) -> (20.1309, 8.1308)
  line L144 (20.1309, 8.1308) -> (19.6069, 8.1308)
  line L145 (19.6069, 8.1308) -> (19.0533, 9.4358)
  line L146 (19.0533, 9.4358) -> (19.0533, 7.414)
  line L147 (19.0533, 7.414) -> (18.3315, 7.414)
  line L148 (18.3315, 7.414) -> (18.3315, 10.464)
  line L149 (18.3315, 10.464) -> (19.2139, 10.464)
  line L150 (19.2139, 10.464) -> (19.8911, 8.9588)
  line L151 (19.8911, 8.9588) -> (20.5634, 10.464)
  line L152 (20.5634, 10.464) -> (21.4458, 10.464)
  line L153 (21.4458, 10.464) -> (21.4458, 7.414)
  line L154 (24.3129, 7.414) -> (22.0711, 7.414)
  line L155 (22.0711, 7.414) -> (22.0711, 7.9108)
  spline S116 degree 2 poles (22.0711, 7.9108) (22.3554, 8.1382) (22.8101, 8.5386) (22.9807, 8.719) knots 0 0 0 1 2 2 2
  spline S117 degree 2 poles (22.9807, 8.719) (23.2056, 8.9538) (23.4058, 9.3122) (23.4058, 9.5001) knots 0 0 0 1 2 2 2
  spline S118 degree 2 poles (23.4058, 9.5001) (23.4058, 9.7126) (23.1512, 9.94) (22.9238, 9.94) knots 0 0 0 1 2 2 2
  spline S119 degree 2 poles (22.9238, 9.94) (22.8077, 9.94) (22.6001, 9.8832) (22.4938, 9.8387) knots 0 0 0 1 2 2 2
  spline S120 degree 2 poles (22.4938, 9.8387) (22.39, 9.7917) (22.2417, 9.6928) (22.2046, 9.6681) knots 0 0 0 1 2 2 2
  line L156 (22.2046, 9.6681) -> (22.1453, 9.6681)
  line L157 (22.1453, 9.6681) -> (22.1453, 10.333)
  spline S121 degree 2 poles (22.1453, 10.333) (22.2738, 10.3948) (22.8225, 10.5233) (23.0771, 10.5233) knots 0 0 0 1 2 2 2
  spline S122 degree 2 poles (23.0771, 10.5233) (23.6208, 10.5233) (24.1794, 10.0389) (24.1794, 9.6014) knots 0 0 0 1 2 2 2
  spline S123 degree 2 poles (24.1794, 9.6014) (24.1794, 9.332) (23.9248, 8.8129) (23.6307, 8.5163) knots 0 0 0 1 2 2 2
  spline S124 degree 2 poles (23.6307, 8.5163) (23.4454, 8.3334) (23.0969, 8.0492) (23.0202, 7.9899) knots 0 0 0 1 2 2 2
  line L158 (23.0202, 7.9899) -> (24.3129, 7.9899)
  line L159 (24.3129, 7.9899) -> (24.3129, 7.414)
  spline S125 degree 2 poles (26.9155, 8.4471) (26.9155, 8.2074) (26.7524, 7.802) (26.5917, 7.6562) knots 0 0 0 1 2 2 2
  spline S126 degree 2 poles (26.5917, 7.6562) (26.4311, 7.5104) (25.9911, 7.3497) (25.6698, 7.3497) knots 0 0 0 1 2 2 2
  spline S127 degree 2 poles (25.6698, 7.3497) (25.3287, 7.3522) (24.8394, 7.4634) (24.6787, 7.5351) knots 0 0 0 1 2 2 2
  line L160 (24.6787, 7.5351) -> (24.6787, 8.2)
  line L161 (24.6787, 8.2) -> (24.7479, 8.2)
  spline S128 degree 2 poles (24.7479, 8.2) (24.8072, 8.1678) (24.9506, 8.0838) (25.0667, 8.0393) knots 0 0 0 1 2 2 2
  spline S129 degree 2 poles (25.0667, 8.0393) (25.1755, 7.9973) (25.4004, 7.9405) (25.5364, 7.9405) knots 0 0 0 1 2 2 2
  spline S130 degree 2 poles (25.5364, 7.9405) (25.655, 7.9405) (25.9318, 7.9998) (26.0159, 8.0789) knots 0 0 0 1 2 2 2
  spline S131 degree 2 poles (26.0159, 8.0789) (26.0776, 8.1407) (26.1469, 8.2914) (26.1469, 8.4175) knots 0 0 0 1 2 2 2
  spline S132 degree 2 poles (26.1469, 8.4175) (26.1469, 8.5262) (26.0579, 8.6795) (25.9862, 8.7264) knots 0 0 0 1 2 2 2
  spline S133 degree 2 poles (25.9862, 8.7264) (25.8824, 8.7956) (25.5858, 8.8352) (25.4795, 8.8352) knots 0 0 0 1 2 2 2
  spline S134 degree 2 poles (25.4795, 8.8352) (25.3114, 8.8352) (24.9926, 8.7808) (24.8764, 8.7511) knots 0 0 0 1 2 2 2
  line L162 (24.8764, 8.7511) -> (24.8097, 8.7511)
  line L163 (24.8097, 8.7511) -> (24.8097, 10.464)
  line L164 (24.8097, 10.464) -> (26.8315, 10.464)
  line L165 (26.8315, 10.464) -> (26.8315, 9.8881)
  line L166 (26.8315, 9.8881) -> (25.5339, 9.8881)
  line L167 (25.5339, 9.8881) -> (25.5339, 9.3814)
  spline S135 degree 2 poles (25.5339, 9.3814) (25.5957, 9.3864) (25.7662, 9.3913) (25.8132, 9.3913) knots 0 0 0 1 2 2 2
  spline S136 degree 2 poles (25.8132, 9.3913) (26.0332, 9.3913) (26.4039, 9.3023) (26.5497, 9.2109) knots 0 0 0 1 2 2 2
  spline S137 degree 2 poles (26.5497, 9.2109) (26.7227, 9.0972) (26.9155, 8.719) (26.9155, 8.4471) knots 0 0 0 1 2 2 2
  spline S138 degree 2 poles (29.5775, 9.1095) (29.5775, 8.7215) (29.3971, 8.0739) (29.2067, 7.8416) knots 0 0 0 1 2 2 2
  spline S139 degree 2 poles (29.2067, 7.8416) (29.009, 7.6068) (28.4257, 7.3547) (28.0006, 7.3547) knots 0 0 0 1 2 2 2
  spline S140 degree 2 poles (28.0006, 7.3547) (27.8572, 7.3547) (27.5458, 7.3917) (27.4939, 7.4066) knots 0 0 0 1 2 2 2
  line L168 (27.4939, 7.4066) -> (27.4939, 8.0047)
  line L169 (27.4939, 8.0047) -> (27.5532, 8.0047)
  spline S141 degree 2 poles (27.5532, 8.0047) (27.6101, 7.9751) (27.8226, 7.9108) (28.008, 7.9108) knots 0 0 0 1 2 2 2
  spline S142 degree 2 poles (28.008, 7.9108) (28.1588, 7.9108) (28.4381, 7.9899) (28.5369, 8.0764) knots 0 0 0 1 2 2 2
  spline S143 degree 2 poles (28.5369, 8.0764) (28.6432, 8.1678) (28.7816, 8.4373) (28.8063, 8.6399) knots 0 0 0 1 2 2 2
  spline S144 degree 2 poles (28.8063, 8.6399) (28.6432, 8.5386) (28.3614, 8.4298) (28.1513, 8.4298) knots 0 0 0 1 2 2 2
  spline S145 degree 2 poles (28.1513, 8.4298) (27.9956, 8.4298) (27.7065, 8.5139) (27.5878, 8.6029) knots 0 0 0 1 2 2 2
  spline S146 degree 2 poles (27.5878, 8.6029) (27.4296, 8.724) (27.2443, 9.112) (27.2443, 9.4185) knots 0 0 0 1 2 2 2
  spline S147 degree 2 poles (27.2443, 9.4185) (27.2443, 9.6582) (27.4074, 10.0611) (27.5557, 10.2094) knots 0 0 0 1 2 2 2
  spline S148 degree 2 poles (27.5557, 10.2094) (27.704, 10.3577) (28.134, 10.5258) (28.3985, 10.5258) knots 0 0 0 1 2 2 2
  spline S149 degree 2 poles (28.3985, 10.5258) (28.6654, 10.5258) (29.0782, 10.3775) (29.2265, 10.2218) knots 0 0 0 1 2 2 2
  spline S150 degree 2 poles (29.2265, 10.2218) (29.3995, 10.0488) (29.5775, 9.5001) (29.5775, 9.1095) knots 0 0 0 1 2 2 2
  spline S151 degree 2 poles (28.8187, 9.2232) (28.8187, 9.4729) (28.7347, 9.7942) (28.658, 9.8832) knots 0 0 0 1 2 2 2
  spline S152 degree 2 poles (28.658, 9.8832) (28.6061, 9.9499) (28.4727, 10.0067) (28.396, 10.0067) knots 0 0 0 1 2 2 2
  spline S153 degree 2 poles (28.396, 10.0067) (28.3268, 10.0067) (28.1983, 9.9524) (28.139, 9.8832) knots 0 0 0 1 2 2 2
  spline S154 degree 2 poles (28.139, 9.8832) (28.0871, 9.8238) (28.0129, 9.594) (28.0129, 9.458) knots 0 0 0 1 2 2 2
  spline S155 degree 2 poles (28.0129, 9.458) (28.0129, 9.3097) (28.0896, 9.1194) (28.1538, 9.0626) knots 0 0 0 1 2 2 2
  spline S156 degree 2 poles (28.1538, 9.0626) (28.2206, 9.0057) (28.3862, 8.9612) (28.49, 8.9612) knots 0 0 0 1 2 2 2
  spline S157 degree 2 poles (28.49, 8.9612) (28.5765, 8.9612) (28.7569, 9.0082) (28.8137, 9.0329) knots 0 0 0 1 2 2 2
  spline S158 degree 2 poles (28.8137, 9.0329) (28.8137, 9.0552) (28.8187, 9.1392) (28.8187, 9.2232) knots 0 0 0 1 2 2 2
  spline S159 degree 2 poles (32.3111, 8.4521) (32.3111, 7.9701) (31.7006, 7.3497) (31.1667, 7.3497) knots 0 0 0 1 2 2 2
  spline S160 degree 2 poles (31.1667, 7.3497) (30.8998, 7.3497) (30.4821, 7.503) (30.3363, 7.6537) knots 0 0 0 1 2 2 2
  spline S161 degree 2 poles (30.3363, 7.6537) (30.1633, 7.8292) (29.9779, 8.3853) (29.9779, 8.7734) knots 0 0 0 1 2 2 2
  spline S162 degree 2 poles (29.9779, 8.7734) (29.9779, 9.1738) (30.1509, 9.7967) (30.3462, 10.0364) knots 0 0 0 1 2 2 2
  spline S163 degree 2 poles (30.3462, 10.0364) (30.5315, 10.2638) (31.1346, 10.5208) (31.5474, 10.5208) knots 0 0 0 1 2 2 2
  spline S164 degree 2 poles (31.5474, 10.5208) (31.6981, 10.5208) (31.9997, 10.4813) (32.0541, 10.4689) knots 0 0 0 1 2 2 2
  line L170 (32.0541, 10.4689) -> (32.0541, 9.8708)
  line L171 (32.0541, 9.8708) -> (31.9997, 9.8708)
  spline S165 degree 2 poles (31.9997, 9.8708) (31.9453, 9.898) (31.6981, 9.9647) (31.54, 9.9647) knots 0 0 0 1 2 2 2
  spline S166 degree 2 poles (31.54, 9.9647) (31.1816, 9.9647) (30.7911, 9.5866) (30.7441, 9.2356) knots 0 0 0 1 2 2 2
  spline S167 degree 2 poles (30.7441, 9.2356) (30.8949, 9.332) (31.2038, 9.4457) (31.3991, 9.4457) knots 0 0 0 1 2 2 2
  spline S168 degree 2 poles (31.3991, 9.4457) (31.5647, 9.4457) (31.8539, 9.3567) (31.9651, 9.2727) knots 0 0 0 1 2 2 2
  spline S169 degree 2 poles (31.9651, 9.2727) (32.1233, 9.1516) (32.3111, 8.7586) (32.3111, 8.4521) knots 0 0 0 1 2 2 2
  spline S170 degree 2 poles (31.4189, 7.9924) (31.4782, 8.0665) (31.5424, 8.2395) (31.5424, 8.415) knots 0 0 0 1 2 2 2
  spline S171 degree 2 poles (31.5424, 8.415) (31.5424, 8.5633) (31.4683, 8.7561) (31.4016, 8.8129) knots 0 0 0 1 2 2 2
  spline S172 degree 2 poles (31.4016, 8.8129) (31.3323, 8.8723) (31.1618, 8.9143) (31.0654, 8.9143) knots 0 0 0 1 2 2 2
  spline S173 degree 2 poles (31.0654, 8.9143) (30.9838, 8.9143) (30.8158, 8.8723) (30.7416, 8.8426) knots 0 0 0 1 2 2 2
  spline S174 degree 2 poles (30.7416, 8.8426) (30.7416, 8.8228) (30.7367, 8.7289) (30.7367, 8.6572) knots 0 0 0 1 2 2 2
  spline S175 degree 2 poles (30.7367, 8.6572) (30.7367, 8.3928) (30.8281, 8.0739) (30.8998, 7.9924) knots 0 0 0 1 2 2 2
  spline S176 degree 2 poles (30.8998, 7.9924) (30.9517, 7.9256) (31.0901, 7.8688) (31.1643, 7.8688) knots 0 0 0 1 2 2 2
  spline S177 degree 2 poles (31.1643, 7.8688) (31.2261, 7.8688) (31.3694, 7.9306) (31.4189, 7.9924) knots 0 0 0 1 2 2 2
  line L172 (15.8451, 2.3922) -> (13.6033, 2.3922)
  line L173 (13.6033, 2.3922) -> (13.6033, 2.889)
  spline S178 degree 2 poles (13.6033, 2.889) (13.8875, 3.1164) (14.3423, 3.5168) (14.5129, 3.6973) knots 0 0 0 1 2 2 2
  spline S179 degree 2 poles (14.5129, 3.6973) (14.7378, 3.9321) (14.938, 4.2905) (14.938, 4.4783) knots 0 0 0 1 2 2 2